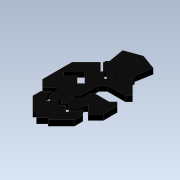
# Autodesk Inventor part: New Logo
Saved by Autodesk Inventor 2020 (Build 240168000, 168)
## iProperties
Created: 2021-10-28
Part Number: New Logo
Material: Generic
Document SubType Name: Modeling
Designer: Turing
Density: 1 g/cm^3
Appearance: Black Control Joints
Author: Turing
Autodesk Inventor part; units mm, degrees
ref_plane "YZ Plane" through (0, 0, 0) normal (1, 0, 0) x (0, 1, 0)
ref_plane "XZ Plane" through (0, 0, 0) normal (0, 1, 0) x (-1, 0, 0)
ref_plane "XY Plane" through (0, 0, 0) normal (0, 0, 1) x (1, 0, 0)
sketch "Sketch1" plane through (0, 0, 0) normal (0, 1, 0) x (-1, 0, 0)
  line L0 (0, 0) -> (-7.0711, -7.0711)
  line L1 (0, 0) -> (7.0711, -7.0711)
  line L2 (0, 0) -> (-1, 0)
  line L3 (7.0711, -7.0711) -> (17.6777, 3.5355)
  line L4 (-7.0711, -7.0711) -> (-17.6777, 3.5355)
  line L5 (0, 0) -> (0, 5)
  line L6 (0, 5) -> (7.0711, -2.0711)
  line L7 (7.0711, -2.0711) -> (17.6777, 8.5355)
  line L8 (0, 5) -> (-7.0711, -2.0711)
  line L9 (-7.0711, -2.0711) -> (-17.6777, 8.5355)
  line L10 (17.6777, 3.5355) -> (24.7487, -3.5355)
  line L11 (-17.6777, 3.5355) -> (-24.7487, -3.5355)
  line L12 (17.6777, 8.5355) -> (28.2843, -2.0711)
  line L13 (-17.6777, 8.5355) -> (-28.2843, -2.0711)
  line L14 (24.7487, -3.5355) -> (24.7487, -18.5355)
  line L15 (-24.7487, -3.5355) -> (-24.7487, -18.5355)
  line L16 (28.2843, -2.0711) -> (28.2843, -12.0711)
  line L17 (-28.2843, -2.0711) -> (-28.2843, -12.0711)
  line L18 (28.2843, -12.0711) -> (38.8909, -1.4645)
  line L19 (-28.2843, -12.0711) -> (-38.8909, -1.4645)
  line L20 (38.8909, -1.4645) -> (38.8909, 13.5355)
  line L21 (38.8909, 13.5355) -> (17.6777, 34.7487)
  line L22 (-38.8909, -1.4645) -> (-38.8909, 13.5355)
  line L23 (-38.8909, 13.5355) -> (-17.6777, 34.7487)
  line L24 (-17.6777, 34.7487) -> (17.6777, 34.7487)
  line L25 (24.7487, -18.5355) -> (28.2843, -22.0711)
  line L26 (28.2843, -22.0711) -> (42.4264, -7.9289)
  line L27 (-24.7487, -18.5355) -> (-28.2843, -22.0711)
  line L28 (-28.2843, -22.0711) -> (-42.4264, -7.9289)
  line L29 (17.6777, 34.7487) -> (14.1421, 38.2843)
  line L30 (14.1421, 38.2843) -> (10.6066, 34.7487)
  line L31 (0, 34.7487) -> (0, 45.7487)
  line L32 (10.6066, 34.7487) -> (0, 34.7487)
  line L33 (5.3033, 34.7487) -> (0, 34.7487)
  line L34 (0, 45.7487) -> (10.6066, 34.7487)
  line L35 (-17.6777, 34.7487) -> (-14.1421, 38.2843)
  line L36 (-14.1421, 38.2843) -> (-10.6066, 34.7487)
  line L37 (0, 45.7487) -> (-10.6066, 34.7487)
  line L38 (-42.4264, -7.9289) -> (-56.5685, -22.0711)
  line L39 (42.4264, -7.9289) -> (56.5685, -22.0711)
  line L40 (0, 0) -> (0, -18.5355)
  line L41 (0, -18.5355) -> (-10.6066, -29.1421)
  line L42 (-10.6066, -29.1421) -> (-10.6066, -44.1421)
  line L43 (-10.6066, -44.1421) -> (-14.1421, -47.6777)
  line L44 (-56.5685, -22.0711) -> (-56.5685, -47.6777)
  line L45 (-14.1421, -47.6777) -> (-56.5685, -47.6777)
  line L46 (-56.5685, -47.6777) -> (-49.4975, -54.7487)
  line L47 (-49.4975, -54.7487) -> (-42.4264, -47.6777)
  line L48 (-56.5685, -47.6777) -> (-52.6777, -47.6777)
  line L49 (-47.6777, -47.6777) -> (-42.4264, -47.6777)
  line L50 (-10.6066, -36.8853) -> (-5.6066, -36.8853)
  line L51 (-6.1919, -24.7274) -> (-2.6564, -28.263)
  line L52 (-5.6066, -36.8853) -> (-5.6066, -31.2132)
  line L53 (-5.6066, -31.2132) -> (-2.6564, -28.263)
  line L54 (0, -18.5355) -> (0, -25.6066)
  line L55 (0, -25.6066) -> (-2.6564, -28.263)
  line L56 (-5.6066, -36.8853) -> (-5.6066, -44.1422)
  line L57 (-5.6066, -44.1422) -> (-5.6066, -64.1422)
  line L58 (-5.6066, -64.1422) -> (-14.1421, -72.6777)
  line L59 (-14.1421, -72.6777) -> (-46.6651, -72.6777)
  line L60 (-46.6651, -72.6777) -> (-53.6117, -79.6243)
  line L61 (56.5685, -22.0711) -> (56.5685, -47.6777)
  line L62 (42.4264, -7.9289) -> (42.4264, -47.6786)
  line L63 (17.6777, 3.5355) -> (17.6777, -47.6786)
  line L64 (17.6777, -47.6786) -> (10.6066, -54.7497)
  line L65 (42.4264, -47.6786) -> (49.4975, -54.7497)
  line L66 (17.6777, -47.6786) -> (30.052, -60.053)
  line L67 (30.052, -60.053) -> (42.4264, -47.6786)
  line L68 (10.6066, -54.7497) -> (30.052, -74.1951)
  line L69 (30.052, -74.1951) -> (49.4975, -54.7497)
  line L70 (56.5685, -47.6777) -> (56.5685, -76.6674)
  line L71 (0, -25.6066) -> (0, -125.6066)
  line L72 (56.5685, -76.6674) -> (30.052, -103.1839)
  line L73 (30.052, -103.1839) -> (30.052, -74.1951)
  line L74 (30.052, -103.1839) -> (0, -103.1839)
  line L75 (0, -103.1839) -> (-30.052, -103.1839)
  line L76 (-53.6117, -79.6243) -> (-30.052, -103.1839)
  line L77 (30.052, -103.1839) -> (0, -73.1319)
  line L78 (-30.052, -103.1839) -> (0, -73.1319)
  line L79 (0, -73.1319) -> (0, -88.1319)
  line L80 (15.026, -88.1579) -> (11.4905, -91.6934)
  line L81 (11.4905, -91.6934) -> (0, -80.2029)
  line L82 (0, -80.2029) -> (-11.4905, -91.6934)
  line L83 (-11.4905, -91.6934) -> (-15.026, -88.1579)
  line L84 (0, -80.2029) -> (0, -85.2029)
  line L85 (0, -85.2029) -> (10.6066, -95.8095)
  line L86 (0, -85.2029) -> (-10.6066, -95.8095)
  line L87 (-10.6066, -95.8095) -> (-14.1421, -92.274)
  line L88 (10.6066, -95.8095) -> (14.1421, -92.274)
  line L89 (14.1421, -92.274) -> (26.87, -105.002)
  line L90 (-14.1421, -92.274) -> (-26.87, -105.002)
  line L91 (-26.87, -105.002) -> (-26.87, -110.002)
  line L92 (26.87, -105.002) -> (26.87, -110.002)
  line L93 (-26.87, -105.002) -> (-30.052, -105.002)
  line L94 (26.87, -110.002) -> (23.3345, -113.5375)
  line L95 (-26.87, -110.002) -> (-23.3345, -113.5375)
  line L96 (23.3345, -113.5375) -> (-23.3345, -113.5375)
  line L97 (0, -113.5375) -> (23.3345, -113.5375)
  line L98 (0, -113.5375) -> (-23.3345, -113.5375)
  line L99 (23.3345, -113.5375) -> (28.5439, -143.0817)
  line L100 (28.5439, -143.0817) -> (-1.5262, -154.0264)
  line L101 (-23.3345, -113.5375) -> (-28.5439, -143.0817)
  line L102 (-28.5439, -143.0817) -> (1.5262, -154.0264)
  line L103 (1.5262, -154.0264) -> (-1.5262, -154.0264)
  point P0 (0, -153.4709)
  dimension "d0" = 10
  dimension "d1" = 90
  dimension "d2" = 45
  dimension "d3" = 1
  dimension "d4" = 15
  dimension "d5" = 90
  dimension "d6" = 10
  dimension "d7" = 15
  dimension "d8" = 90
  dimension "d9" = 5
  dimension "d10" = 10
  dimension "d11" = 45
  dimension "d12" = 15
  dimension "d13" = 10
  dimension "d14" = 45
  dimension "d15" = 15
  dimension "d16" = 90
  dimension "d17" = 10
  dimension "d18" = 90
  dimension "d19" = 10
  dimension "d20" = 90
  dimension "d21" = 15
  dimension "d22" = 90
  dimension "d23" = 15
  dimension "d24" = 90
  dimension "d25" = 15
  dimension "d26" = 15
  dimension "d27" = 10
  dimension "d28" = 15
  dimension "d29" = 45
  dimension "d30" = 15
  dimension "d31" = 45
  dimension "d32" = 10
  dimension "d33" = 15
  dimension "d34" = 135
  dimension "d35" = 30
  dimension "d36" = 30
  dimension "d37" = 135
  dimension "d38" = 5
  dimension "d39" = 135
  dimension "d40" = 90
  dimension "d41" = 20
  dimension "d42" = 5
  dimension "d43" = 20
  dimension "d44" = 135
  dimension "d45" = 5
  dimension "d46" = 11
  dimension "d47" = 5
  dimension "d48" = 45
  dimension "d49" = 5
  dimension "d50" = 90
  dimension "d51" = 20
  dimension "d52" = 20
  dimension "d53" = 90
  dimension "d54" = 15
  dimension "d55" = 15
  dimension "d56" = 5
  dimension "d57" = 135
  dimension "d58" = 18.5355
  dimension "d59" = 10
  dimension "d60" = 10
  dimension "d61" = 45
  dimension "d62" = 45
  dimension "d63" = 3.8909
  constraints: 208 end point, 18 vertical, 16 point on line, 13 perpendicular, 8 horizontal, 5 collinear, 5 midpoint, 3 parallel
  measures "d0" distance of L0.start L0.end
  measures "d1" angle of L0 L1
  measures "d2" angle of L0 L2
  measures "d3" distance of L0.start L2.end
  measures "d4" distance of L1.end L3.end
  measures "d5" angle of L1 L3
  measures "d6" distance of L0.start L1.end
  measures "d7" distance of L0.end L4.end
  measures "d8" angle of L4 L0
  measures "d9" distance of L0.start L5.end
  measures "d10" distance of L5.end L6.end
  measures "d11" angle of L5 L6
  measures "d12" distance of L6.end L7.end
  measures "d13" distance of L5.end L8.end
  measures "d14" angle of L5 L8
  measures "d15" distance of L8.end L9.end
  measures "d16" angle of L6 L7
  measures "d17" distance of L3.end L10.end
  measures "d18" angle of L3 L10
  measures "d19" distance of L4.end L11.end
  measures "d20" angle of L11 L4
  measures "d21" distance of L7.end L12.end
  measures "d22" angle of L7 L12
  measures "d23" distance of L9.end L13.end
  measures "d24" angle of L13 L9
  measures "d25" distance of L10.end L14.end
  measures "d26" distance of L11.end L15.end
  measures "d27" distance of L12.end L16.end
  measures "d28" distance of L16.end L18.end
  measures "d29" angle of L16 L18
  measures "d30" distance of L17.end L19.end
  measures "d31" angle of L19 L17
  measures "d32" distance of L13.end L17.end
  measures "d33" distance of L18.end L20.end
  measures "d34" angle of L20 L21
  measures "d35" distance of L20.end L21.end
  measures "d36" distance of L22.end L23.end
  measures "d37" angle of L22 L23
  measures "d38" distance of L14.end L25.end
  measures "d39" angle of L25 L14
  measures "d40" angle of L25 L26
  measures "d41" distance of L25.end L26.end
  measures "d42" distance of L15.end L27.end
  measures "d43" distance of L27.end L28.end
  measures "d44" angle of L15 L27
  measures "d45" distance of L21.end L29.end
  measures "d46" distance of L31.start L31.end
  measures "d47" distance of L23.end L35.end
  measures "d48" angle of L24 L35
  measures "d49" distance of L35.end L36.end
  measures "d50" angle of L38 L28
  measures "d51" distance of L28.end L38.end
  measures "d52" distance of L26.end L39.end
  measures "d53" angle of L26 L39
  measures "d54" distance of L40.end L41.end
  measures "d55" distance of L41.end L42.end
  measures "d56" distance of L42.end L43.end
  measures "d57" angle of L42 L41
  measures "d58" distance of L0.start L40.end
  measures "d59" distance of L46.end L47.end
  measures "d60" distance of L44.end L46.end
  measures "d61" angle of L49 L47
  measures "d62" angle of L46 L45
  measures "d63" distance of L48.end L44.end
extrude "Extrusion1" add sketch "Sketch1" along normal blind 10 contours L40 L41 L42 L43 L45 L44 L38 L28 L27 L15 L11 L4 L0 | L1 L3 L63 L64 L68 L73 L77 L71 L54 L40 | L10 L14 L25 L26 L62 L67 L66 L63 | L71 L78 L76 L60 L59 L58 L57 L56 L52 L53 L55 | L77 L80 L81 L71 | L71 L82 L83 L78 | L69 L65 L62 L39 L61 L70 L72 L73 | L85 L88 L89 L74 L71 | L71 L75 L90 L87 L86 | L89 L92 L94 L96 L71 L74 | L75 L71 L96 L95 L91 L90 | L47 L46 L45 | L96 L99 L100 L102 L101 | L8 L9 L13 L17 L19 L22 L23 L24 L21 L20 L18 L16 L12 L7 L6 | L24 L30 L29 | L35 L36 L24 | L24 L31 L34 | L37 L31 L24
equation "\"d4\" = d7"
equation "\"d5\" = d1"
equation "\"d6\" = d0"
equation "\"d7\" = 1.5 * d0"
equation "\"d8\" = d1"
equation "\"d10\" = d0"
equation "\"d11\" = d2"
equation "\"d12\" = d7"
equation "\"d13\" = d0"
equation "\"d14\" = d2"
equation "\"d15\" = d7"
equation "\"d16\" = d1"
equation "\"d18\" = d1"
equation "\"d20\" = d1"
equation "\"d21\" = d7"
equation "\"d22\" = d1"
equation "\"d23\" = d7"
equation "\"d24\" = d1"
equation "\"d25\" = d7"
equation "\"d26\" = d7"
equation "\"d27\" = d0"
equation "\"d28\" = d7"
equation "\"d29\" = d2"
equation "\"d30\" = d7"
equation "\"d31\" = d2"
equation "\"d32\" = d0"
equation "\"d33\" = d7"
equation "\"d36\" = d35"
equation "\"d37\" = d34"
equation "\"d38\" = 0.5 * d0"
equation "\"d41\" = 2 * d0"
equation "\"d42\" = d38"
equation "\"d43\" = d41"
equation "\"d44\" = d39"
equation "\"d47\" = d45"
equation "\"d50\" = d1"
equation "\"d51\" = d43"
equation "\"d52\" = d43"
equation "\"d53\" = d1"
body "Solid1"
